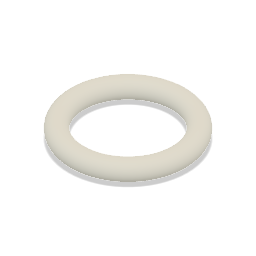
玉环 v2 (Autodesk Fusion 360 design; units mm, degrees)
Autodesk Fusion 360 part; units mm, degrees
torus "圆环体基本要素1" add centre line diameter 110 section diameter 20 placed x (1, 0, 0) y (0, 0, -1) z (0, 1, 0) at (-50, 0, 0)
